Autodesk Inventor part; units mm, degrees
(part 3 of 3)
  line L456 (12.9282, 16.8333) -> (13.3502, 16.5006)
  line L457 (13.3502, 16.5006) -> (13.3076, 16.2984)
  line L458 (13.3076, 16.2984) -> (13.2446, 16.0331)
  line L459 (13.2446, 16.0331) -> (13.1744, 15.773)
  line L460 (13.1744, 15.773) -> (13.0968, 15.5182)
  line L461 (13.0968, 15.5182) -> (13.0115, 15.2694)
  line L462 (13.0115, 15.2694) -> (12.9181, 15.0268)
  line L463 (12.9181, 15.0268) -> (12.8161, 14.7913)
  line L464 (12.8161, 14.7913) -> (12.7045, 14.5637)
  line L465 (12.7045, 14.5637) -> (12.6447, 14.4533)
  line L466 (12.6447, 14.4533) -> (12.5818, 14.3456)
  line L467 (12.5818, 14.3456) -> (12.5153, 14.241)
  line L468 (12.5153, 14.241) -> (12.4803, 14.1901)
  line L469 (12.4803, 14.1901) -> (12.4439, 14.1406)
  line L470 (12.4439, 14.1406) -> (12.6143, 13.9062)
  line L471 (12.6143, 13.9062) -> (12.8737, 13.6665)
  line L472 (12.8737, 13.6665) -> (13.1207, 13.515)
  line L473 (13.1207, 13.515) -> (13.1672, 13.5552)
  line L474 (13.1672, 13.5552) -> (13.2151, 13.594)
  line L475 (13.2151, 13.594) -> (13.3142, 13.6686)
  line L476 (13.3142, 13.6686) -> (13.4166, 13.7397)
  line L477 (13.4166, 13.7397) -> (13.522, 13.808)
  line L478 (13.522, 13.808) -> (13.7402, 13.9371)
  line L479 (13.7402, 13.9371) -> (13.967, 14.0573)
  line L480 (13.967, 14.0573) -> (14.2014, 14.1694)
  line L481 (14.2014, 14.1694) -> (14.4428, 14.274)
  line L482 (14.4428, 14.274) -> (14.6907, 14.3714)
  line L483 (14.6907, 14.3714) -> (14.9445, 14.4617)
  line L484 (14.9445, 14.4617) -> (15.2041, 14.5453)
  line L485 (15.2041, 14.5453) -> (15.4023, 14.6036)
  line L486 (15.4023, 14.6036) -> (15.7671, 14.209)
  line L487 (15.7671, 14.209) -> (15.6934, 14.016)
  line L488 (15.6934, 14.016) -> (15.5897, 13.7638)
  line L489 (15.5897, 13.7638) -> (15.4797, 13.5178)
  line L490 (15.4797, 13.5178) -> (15.3632, 13.2784)
  line L491 (15.3632, 13.2784) -> (15.24, 13.0459)
  line L492 (15.24, 13.0459) -> (15.1098, 12.821)
  line L493 (15.1098, 12.821) -> (14.9722, 12.6043)
  line L494 (14.9722, 12.6043) -> (14.8264, 12.397)
  line L495 (14.8264, 12.397) -> (14.75, 12.2973)
  line L496 (14.75, 12.2973) -> (14.671, 12.2007)
  line L497 (14.671, 12.2007) -> (14.589, 12.1078)
  line L498 (14.589, 12.1078) -> (14.5465, 12.0631)
  line L499 (14.5465, 12.0631) -> (14.5028, 12.0199)
  line L500 (14.5028, 12.0199) -> (14.6344, 11.7617)
  line L501 (14.6344, 11.7617) -> (14.8531, 11.4843)
  line L502 (14.8531, 11.4843) -> (15.0734, 11.2961)
  line L503 (15.0734, 11.2961) -> (15.1256, 11.3285)
  line L504 (15.1256, 11.3285) -> (15.179, 11.3594)
  line L505 (15.179, 11.3594) -> (15.2885, 11.4175)
  line L506 (15.2885, 11.4175) -> (15.4008, 11.4717)
  line L507 (15.4008, 11.4717) -> (15.5156, 11.5227)
  line L508 (15.5156, 11.5227) -> (15.7512, 11.6161)
  line L509 (15.7512, 11.6161) -> (15.9941, 11.6993)
  line L510 (15.9941, 11.6993) -> (16.2432, 11.7734)
  line L511 (16.2432, 11.7734) -> (16.498, 11.8389)
  line L512 (16.498, 11.8389) -> (16.758, 11.8963)
  line L513 (16.758, 11.8963) -> (17.0229, 11.9459)
  line L514 (17.0229, 11.9459) -> (17.2923, 11.9878)
  line L515 (17.2923, 11.9878) -> (17.4972, 12.0144)
  line L516 (17.4972, 12.0144) -> (17.7957, 11.5676)
  line L517 (17.7957, 11.5676) -> (17.6928, 11.3885)
  line L518 (17.6928, 11.3885) -> (17.5509, 11.1556)
  line L519 (17.5509, 11.1556) -> (17.4037, 10.9299)
  line L520 (17.4037, 10.9299) -> (17.2512, 10.7116)
  line L521 (17.2512, 10.7116) -> (17.0932, 10.5012)
  line L522 (17.0932, 10.5012) -> (16.9294, 10.2995)
  line L523 (16.9294, 10.2995) -> (16.7596, 10.107)
  line L524 (16.7596, 10.107) -> (16.5831, 9.925)
  line L525 (16.5831, 9.925) -> (16.4921, 9.8385)
  line L526 (16.4921, 9.8385) -> (16.399, 9.7554)
  line L527 (16.399, 9.7554) -> (16.3034, 9.6765)
  line L528 (16.3034, 9.6765) -> (16.2545, 9.639)
  line L529 (16.2545, 9.639) -> (16.2045, 9.6031)
  line L530 (16.2045, 9.6031) -> (16.2942, 9.3276)
  line L531 (16.2942, 9.3276) -> (16.4668, 9.0194)
  line L532 (16.4668, 9.0194) -> (16.6549, 8.799)
  line L533 (16.6549, 8.799) -> (16.7115, 8.8229)
  line L534 (16.7115, 8.8229) -> (16.7691, 8.845)
  line L535 (16.7691, 8.845) -> (16.8863, 8.8853)
  line L536 (16.8863, 8.8853) -> (17.0058, 8.9213)
  line L537 (17.0058, 8.9213) -> (17.1271, 8.9537)
  line L538 (17.1271, 8.9537) -> (17.3745, 9.009)
  line L539 (17.3745, 9.009) -> (17.6273, 9.0533)
  line L540 (17.6273, 9.0533) -> (17.885, 9.0875)
  line L541 (17.885, 9.0875) -> (18.1469, 9.1123)
  line L542 (18.1469, 9.1123) -> (18.4127, 9.1283)
  line L543 (18.4127, 9.1283) -> (18.682, 9.1358)
  line L544 (18.682, 9.1358) -> (18.9547, 9.1351)
  line L545 (18.9547, 9.1351) -> (19.1612, 9.1293)
  line L546 (19.1612, 9.1293) -> (19.3862, 8.6413)
  line L547 (19.3862, 8.6413) -> (19.2565, 8.4805)
  line L548 (19.2565, 8.4805) -> (19.0799, 8.2727)
  line L549 (19.0799, 8.2727) -> (18.8993, 8.0727)
  line L550 (18.8993, 8.0727) -> (18.7145, 7.881)
  line L551 (18.7145, 7.881) -> (18.5255, 7.698)
  line L552 (18.5255, 7.698) -> (18.3322, 7.5243)
  line L553 (18.3322, 7.5243) -> (18.1343, 7.3608)
  line L554 (18.1343, 7.3608) -> (17.9316, 7.2086)
  line L555 (17.9316, 7.2086) -> (17.8282, 7.1374)
  line L556 (17.8282, 7.1374) -> (17.7232, 7.07)
  line L557 (17.7232, 7.07) -> (17.6165, 7.007)
  line L558 (17.6165, 7.007) -> (17.5622, 6.9776)
  line L559 (17.5622, 6.9776) -> (17.5073, 6.95)
  line L560 (17.5073, 6.95) -> (17.5527, 6.6638)
  line L561 (17.5527, 6.6638) -> (17.675, 6.3324)
  line L562 (17.675, 6.3324) -> (17.8263, 6.0853)
  line L563 (17.8263, 6.0853) -> (17.886, 6.1)
  line L564 (17.886, 6.1) -> (17.9463, 6.1128)
  line L565 (17.9463, 6.1128) -> (18.0684, 6.1343)
  line L566 (18.0684, 6.1343) -> (18.192, 6.1512)
  line L567 (18.192, 6.1512) -> (18.3169, 6.1642)
  line L568 (18.3169, 6.1642) -> (18.5699, 6.1802)
  line L569 (18.5699, 6.1802) -> (18.8265, 6.1843)
  line L570 (18.8265, 6.1843) -> (19.0863, 6.1778)
  line L571 (19.0863, 6.1778) -> (19.3489, 6.1613)
  line L572 (19.3489, 6.1613) -> (19.614, 6.1355)
  line L573 (19.614, 6.1355) -> (19.8812, 6.1008)
  line L574 (19.8812, 6.1008) -> (20.1504, 6.0575)
  line L575 (20.1504, 6.0575) -> (20.3535, 6.0194)
  line L576 (20.3535, 6.0194) -> (20.4993, 5.5022)
  line L577 (20.4993, 5.5022) -> (20.346, 5.3637)
  line L578 (20.346, 5.3637) -> (20.1392, 5.1861)
  line L579 (20.1392, 5.1861) -> (19.9295, 5.0169)
  line L580 (19.9295, 5.0169) -> (19.717, 4.8564)
  line L581 (19.717, 4.8564) -> (19.5017, 4.7052)
  line L582 (19.5017, 4.7052) -> (19.2836, 4.5639)
  line L583 (19.2836, 4.5639) -> (19.0626, 4.4333)
  line L584 (19.0626, 4.4333) -> (18.8385, 4.3147)
  line L585 (18.8385, 4.3147) -> (18.7252, 4.2606)
  line L586 (18.7252, 4.2606) -> (18.611, 4.2104)
  line L587 (18.611, 4.2104) -> (18.4957, 4.1649)
  line L588 (18.4957, 4.1649) -> (18.4376, 4.1443)
  line L589 (18.4376, 4.1443) -> (18.379, 4.1257)
  line L590 (18.379, 4.1257) -> (18.3791, 3.8359)
  line L591 (18.3791, 3.8359) -> (18.448, 3.4895)
  line L592 (18.448, 3.4895) -> (18.5588, 3.2217)
  line L593 (18.5588, 3.2217) -> (18.62, 3.2269)
  line L594 (18.62, 3.2269) -> (18.6816, 3.2301)
  line L595 (18.6816, 3.2301) -> (18.8056, 3.2322)
  line L596 (18.8056, 3.2322) -> (18.9303, 3.2296)
  line L597 (18.9303, 3.2296) -> (19.0557, 3.2229)
  line L598 (19.0557, 3.2229) -> (19.3081, 3.1991)
  line L599 (19.3081, 3.1991) -> (19.5622, 3.163)
  line L600 (19.5622, 3.163) -> (19.8178, 3.1159)
  line L601 (19.8178, 3.1159) -> (20.0745, 3.0586)
  line L602 (20.0745, 3.0586) -> (20.3323, 2.9917)
  line L603 (20.3323, 2.9917) -> (20.5908, 2.9156)
  line L604 (20.5908, 2.9156) -> (20.8499, 2.8307)
  line L605 (20.8499, 2.8307) -> (21.0445, 2.7613)
  line L606 (21.0445, 2.7613) -> (21.1077, 2.2277)
  line L607 (21.1077, 2.2277) -> (20.9346, 2.1148)
  line L608 (20.9346, 2.1148) -> (20.7025, 1.9718)
  line L609 (20.7025, 1.9718) -> (20.4689, 1.8374)
  line L610 (20.4689, 1.8374) -> (20.2339, 1.7122)
  line L611 (20.2339, 1.7122) -> (19.9976, 1.5965)
  line L612 (19.9976, 1.5965) -> (19.7601, 1.4911)
  line L613 (19.7601, 1.4911) -> (19.5214, 1.3967)
  line L614 (19.5214, 1.3967) -> (19.2815, 1.3146)
  line L615 (19.2815, 1.3146) -> (19.1612, 1.2789)
  line L616 (19.1612, 1.2789) -> (19.0405, 1.2472)
  line L617 (19.0405, 1.2472) -> (18.9195, 1.2203)
  line L618 (18.9195, 1.2203) -> (18.8589, 1.209)
  line L619 (18.8589, 1.209) -> (18.7981, 1.1998)
  line L620 (18.7981, 1.1998) -> (18.7529, 0.9135)
  line L621 (18.7529, 0.9135) -> (18.7667, 0.5606)
  line L622 (18.7667, 0.5606) -> (18.8343, 0.2788)
  line L623 (18.8343, 0.2788) -> (18.8956, 0.2744)
  line L624 (18.8956, 0.2744) -> (18.9569, 0.2679)
  line L625 (18.9569, 0.2679) -> (19.0797, 0.2506)
  line L626 (19.0797, 0.2506) -> (19.2024, 0.2285)
  line L627 (19.2024, 0.2285) -> (19.3252, 0.2022)
  line L628 (19.3252, 0.2022) -> (19.5708, 0.1393)
  line L629 (19.5708, 0.1393) -> (19.8162, 0.0639)
  line L630 (19.8162, 0.0639) -> (20.0612, -0.0226)
  line L631 (20.0612, -0.0226) -> (20.3059, -0.1194)
  line L632 (20.3059, -0.1194) -> (20.55, -0.2258)
  line L633 (20.55, -0.2258) -> (20.7934, -0.3414)
  line L634 (20.7934, -0.3414) -> (21.036, -0.4658)
  line L635 (21.036, -0.4658) -> (21.2174, -0.5647)
  line L636 (21.2174, -0.5647) -> (21.1963, -1.1017)
  line L637 (21.1963, -1.1017) -> (21.0077, -1.1861)
  line L638 (21.0077, -1.1861) -> (20.7561, -1.2911)
  line L639 (20.7561, -1.2911) -> (20.5043, -1.3872)
  line L640 (20.5043, -1.3872) -> (20.2526, -1.4742)
  line L641 (20.2526, -1.4742) -> (20.0012, -1.5514)
  line L642 (20.0012, -1.5514) -> (19.7501, -1.6184)
  line L643 (19.7501, -1.6184) -> (19.4995, -1.6743)
  line L644 (19.4995, -1.6743) -> (19.2498, -1.7179)
  line L645 (19.2498, -1.7179) -> (19.1253, -1.7343)
  line L646 (19.1253, -1.7343) -> (19.0012, -1.7468)
  line L647 (19.0012, -1.7468) -> (18.8775, -1.7544)
  line L648 (18.8775, -1.7544) -> (18.8158, -1.756)
  line L649 (18.8158, -1.756) -> (18.7543, -1.7557)
  line L650 (18.7543, -1.7557) -> (18.6649, -2.0313)
  line L651 (18.6649, -2.0313) -> (18.6234, -2.3821)
  line L652 (18.6234, -2.3821) -> (18.646, -2.6709)
  line L653 (18.646, -2.6709) -> (18.7059, -2.6849)
  line L654 (18.7059, -2.6849) -> (18.7655, -2.7009)
  line L655 (18.7655, -2.7009) -> (18.884, -2.7372)
  line L656 (18.884, -2.7372) -> (19.0018, -2.7783)
  line L657 (19.0018, -2.7783) -> (19.119, -2.8234)
  line L658 (19.119, -2.8234) -> (19.3516, -2.924)
  line L659 (19.3516, -2.924) -> (19.5822, -3.0368)
  line L660 (19.5822, -3.0368) -> (19.8107, -3.1606)
  line L661 (19.8107, -3.1606) -> (20.0372, -3.2944)
  line L662 (20.0372, -3.2944) -> (20.2616, -3.4377)
  line L663 (20.2616, -3.4377) -> (20.484, -3.59)
  line L664 (20.484, -3.59) -> (20.7042, -3.7508)
  line L665 (20.7042, -3.7508) -> (20.8678, -3.8769)
  line L666 (20.8678, -3.8769) -> (20.763, -4.404)
  line L667 (20.763, -4.404) -> (20.5635, -4.4578)
  line L668 (20.5635, -4.4578) -> (20.2986, -4.5222)
  line L669 (20.2986, -4.5222) -> (20.0349, -4.5777)
  line L670 (20.0349, -4.5777) -> (19.7727, -4.6242)
  line L671 (19.7727, -4.6242) -> (19.5122, -4.6612)
  line L672 (19.5122, -4.6612) -> (19.2537, -4.6881)
  line L673 (19.2537, -4.6881) -> (18.9975, -4.7041)
  line L674 (18.9975, -4.7041) -> (18.7441, -4.708)
  line L675 (18.7441, -4.708) -> (18.6186, -4.7049)
  line L676 (18.6186, -4.7049) -> (18.494, -4.6977)
  line L677 (18.494, -4.6977) -> (18.3706, -4.6859)
  line L678 (18.3706, -4.6859) -> (18.3095, -4.6779)
  line L679 (18.3095, -4.6779) -> (18.2488, -4.6679)
  line L680 (18.2488, -4.6679) -> (18.1173, -4.9261)
  line L681 (18.1173, -4.9261) -> (18.0215, -5.2661)
  line L682 (18.0215, -5.2661) -> (17.9986, -5.5549)
  line L683 (17.9986, -5.5549) -> (18.0556, -5.5781)
  line L684 (18.0556, -5.5781) -> (18.1119, -5.6032)
  line L685 (18.1119, -5.6032) -> (18.2233, -5.6576)
  line L686 (18.2233, -5.6576) -> (18.3332, -5.7166)
  line L687 (18.3332, -5.7166) -> (18.4419, -5.7795)
  line L688 (18.4419, -5.7795) -> (18.656, -5.9153)
  line L689 (18.656, -5.9153) -> (18.866, -6.0628)
  line L690 (18.866, -6.0628) -> (19.0724, -6.2208)
  line L691 (19.0724, -6.2208) -> (19.2751, -6.3884)
  line L692 (19.2751, -6.3884) -> (19.4744, -6.565)
  line L693 (19.4744, -6.565) -> (19.6702, -6.7502)
  line L694 (19.6702, -6.7502) -> (19.8625, -6.9435)
  line L695 (19.8625, -6.9435) -> (20.0044, -7.0936)
  line L696 (20.0044, -7.0936) -> (19.8184, -7.5978)
  line L697 (19.8184, -7.5978) -> (19.613, -7.6198)
  line L698 (19.613, -7.6198) -> (19.3412, -7.6419)
  line L699 (19.3412, -7.6419) -> (19.0721, -7.6555)
  line L700 (19.0721, -7.6555) -> (18.8059, -7.6604)
  line L701 (18.8059, -7.6604) -> (18.5428, -7.6562)
  line L702 (18.5428, -7.6562) -> (18.2833, -7.6423)
  line L703 (18.2833, -7.6423) -> (18.0278, -7.6181)
  line L704 (18.0278, -7.6181) -> (17.7768, -7.5823)
  line L705 (17.7768, -7.5823) -> (17.6533, -7.5595)
  line L706 (17.6533, -7.5595) -> (17.5314, -7.533)
  line L707 (17.5314, -7.533) -> (17.4114, -7.502)
  line L708 (17.4114, -7.502) -> (17.3523, -7.4845)
  line L709 (17.3523, -7.4845) -> (17.2939, -7.4652)
  line L710 (17.2939, -7.4652) -> (17.1237, -7.6996)
  line L711 (17.1237, -7.6996) -> (16.9758, -8.0204)
  line L712 (16.9758, -8.0204) -> (16.908, -8.3021)
  line L713 (16.908, -8.3021) -> (16.9606, -8.334)
  line L714 (16.9606, -8.334) -> (17.0124, -8.3676)
  line L715 (17.0124, -8.3676) -> (17.1139, -8.4387)
  line L716 (17.1139, -8.4387) -> (17.2132, -8.5142)
  line L717 (17.2132, -8.5142) -> (17.3107, -8.5933)
  line L718 (17.3107, -8.5933) -> (17.5009, -8.7609)
  line L719 (17.5009, -8.7609) -> (17.6853, -8.9394)
  line L720 (17.6853, -8.9394) -> (17.8644, -9.1278)
  line L721 (17.8644, -9.1278) -> (18.0385, -9.325)
  line L722 (18.0385, -9.325) -> (18.2076, -9.5307)
  line L723 (18.2076, -9.5307) -> (18.3721, -9.7442)
  line L724 (18.3721, -9.7442) -> (18.5318, -9.9652)
  line L725 (18.5318, -9.9652) -> (18.6484, -10.1357)
  line L726 (18.6484, -10.1357) -> (18.3859, -10.6045)
  line L727 (18.3859, -10.6045) -> (18.1795, -10.5941)
  line L728 (18.1795, -10.5941) -> (17.9077, -10.5734)
  line L729 (17.9077, -10.5734) -> (17.6397, -10.5448)
  line L730 (17.6397, -10.5448) -> (17.376, -10.508)
  line L731 (17.376, -10.508) -> (17.1168, -10.4627)
  line L732 (17.1168, -10.4627) -> (16.8627, -10.4084)
  line L733 (16.8627, -10.4084) -> (16.6141, -10.3444)
  line L734 (16.6141, -10.3444) -> (16.3718, -10.2698)
  line L735 (16.3718, -10.2698) -> (16.2534, -10.228)
  line L736 (16.2534, -10.228) -> (16.1372, -10.1828)
  line L737 (16.1372, -10.1828) -> (16.0235, -10.1334)
  line L738 (16.0235, -10.1334) -> (15.9678, -10.1068)
  line L739 (15.9678, -10.1068) -> (15.9132, -10.0786)
  line L740 (15.9132, -10.0786) -> (15.7083, -10.2836)
  line L741 (15.7083, -10.2836) -> (15.5121, -10.5773)
  line L742 (15.5121, -10.5773) -> (15.4011, -10.8449)
  line L743 (15.4011, -10.8449) -> (15.4481, -10.8846)
  line L744 (15.4481, -10.8846) -> (15.494, -10.9259)
  line L745 (15.494, -10.9259) -> (15.5831, -11.012)
  line L746 (15.5831, -11.012) -> (15.6694, -11.1021)
  line L747 (15.6694, -11.1021) -> (15.7533, -11.1955)
  line L748 (15.7533, -11.1955) -> (15.915, -11.3907)
  line L749 (15.915, -11.3907) -> (16.0692, -11.596)
  line L750 (16.0692, -11.596) -> (16.2166, -11.81)
  line L751 (16.2166, -11.81) -> (16.3576, -12.0321)
  line L752 (16.3576, -12.0321) -> (16.4926, -12.2616)
  line L753 (16.4926, -12.2616) -> (16.6215, -12.4982)
  line L754 (16.6215, -12.4982) -> (16.7447, -12.7415)
  line L755 (16.7447, -12.7415) -> (16.8333, -12.9281)
  line L756 (16.8333, -12.9281) -> (16.5006, -13.3502)
  line L757 (16.5006, -13.3502) -> (16.2984, -13.3076)
  line L758 (16.2984, -13.3076) -> (16.0331, -13.2446)
  line L759 (16.0331, -13.2446) -> (15.773, -13.1744)
  line L760 (15.773, -13.1744) -> (15.5182, -13.0968)
  line L761 (15.5182, -13.0968) -> (15.2694, -13.0115)
  line L762 (15.2694, -13.0115) -> (15.0268, -12.9181)
  line L763 (15.0268, -12.9181) -> (14.7913, -12.8161)
  line L764 (14.7913, -12.8161) -> (14.5637, -12.7045)
  line L765 (14.5637, -12.7045) -> (14.4533, -12.6447)
  line L766 (14.4533, -12.6447) -> (14.3456, -12.5818)
  line L767 (14.3456, -12.5818) -> (14.241, -12.5153)
  line L768 (14.241, -12.5153) -> (14.1901, -12.4803)
  line L769 (14.1901, -12.4803) -> (14.1406, -12.4439)
  line L770 (14.1406, -12.4439) -> (13.9062, -12.6143)
  line L771 (13.9062, -12.6143) -> (13.6665, -12.8737)
  line L772 (13.6665, -12.8737) -> (13.515, -13.1207)
  line L773 (13.515, -13.1207) -> (13.5552, -13.1672)
  line L774 (13.5552, -13.1672) -> (13.594, -13.2151)
  line L775 (13.594, -13.2151) -> (13.6686, -13.3142)
  line L776 (13.6686, -13.3142) -> (13.7397, -13.4166)
  line L777 (13.7397, -13.4166) -> (13.808, -13.522)
  line L778 (13.808, -13.522) -> (13.9371, -13.7402)
  line L779 (13.9371, -13.7402) -> (14.0573, -13.967)
  line L780 (14.0573, -13.967) -> (14.1694, -14.2014)
  line L781 (14.1694, -14.2014) -> (14.274, -14.4428)
  line L782 (14.274, -14.4428) -> (14.3714, -14.6907)
  line L783 (14.3714, -14.6907) -> (14.4617, -14.9445)
  line L784 (14.4617, -14.9445) -> (14.5453, -15.2041)
  line L785 (14.5453, -15.2041) -> (14.6036, -15.4023)
  line L786 (14.6036, -15.4023) -> (14.209, -15.7671)
  line L787 (14.209, -15.7671) -> (14.016, -15.6934)
  line L788 (14.016, -15.6934) -> (13.7638, -15.5897)
  line L789 (13.7638, -15.5897) -> (13.5178, -15.4797)
  line L790 (13.5178, -15.4797) -> (13.2784, -15.3632)
  line L791 (13.2784, -15.3632) -> (13.0459, -15.24)
  line L792 (13.0459, -15.24) -> (12.821, -15.1098)
  line L793 (12.821, -15.1098) -> (12.6043, -14.9722)
  line L794 (12.6043, -14.9722) -> (12.397, -14.8264)
  line L795 (12.397, -14.8264) -> (12.2973, -14.75)
  line L796 (12.2973, -14.75) -> (12.2007, -14.671)
  line L797 (12.2007, -14.671) -> (12.1078, -14.589)
  line L798 (12.1078, -14.589) -> (12.0631, -14.5465)
  line L799 (12.0631, -14.5465) -> (12.0199, -14.5028)
  line L800 (12.0199, -14.5028) -> (11.7617, -14.6344)
  line L801 (11.7617, -14.6344) -> (11.4843, -14.8531)
  line L802 (11.4843, -14.8531) -> (11.2961, -15.0734)
  line L803 (11.2961, -15.0734) -> (11.3285, -15.1256)
  line L804 (11.3285, -15.1256) -> (11.3594, -15.179)
  line L805 (11.3594, -15.179) -> (11.4175, -15.2885)
  line L806 (11.4175, -15.2885) -> (11.4717, -15.4008)
  line L807 (11.4717, -15.4008) -> (11.5227, -15.5156)
  line L808 (11.5227, -15.5156) -> (11.6161, -15.7512)
  line L809 (11.6161, -15.7512) -> (11.6993, -15.9941)
  line L810 (11.6993, -15.9941) -> (11.7734, -16.2432)
  line L811 (11.7734, -16.2432) -> (11.8389, -16.498)
  line L812 (11.8389, -16.498) -> (11.8963, -16.758)
  line L813 (11.8963, -16.758) -> (11.9458, -17.0229)
  line L814 (11.9458, -17.0229) -> (11.9878, -17.2923)
  line L815 (11.9878, -17.2923) -> (12.0144, -17.4972)
  line L816 (12.0144, -17.4972) -> (11.5676, -17.7957)
  line L817 (11.5676, -17.7957) -> (11.3885, -17.6928)
  line L818 (11.3885, -17.6928) -> (11.1556, -17.5509)
  line L819 (11.1556, -17.5509) -> (10.9298, -17.4037)
  line L820 (10.9298, -17.4037) -> (10.7116, -17.2512)
  line L821 (10.7116, -17.2512) -> (10.5012, -17.0932)
  line L822 (10.5012, -17.0932) -> (10.2995, -16.9294)
  line L823 (10.2995, -16.9294) -> (10.107, -16.7596)
  line L824 (10.107, -16.7596) -> (9.925, -16.5831)
  line L825 (9.925, -16.5831) -> (9.8385, -16.4921)
  line L826 (9.8385, -16.4921) -> (9.7554, -16.399)
  line L827 (9.7554, -16.399) -> (9.6765, -16.3034)
  line L828 (9.6765, -16.3034) -> (9.639, -16.2545)
  line L829 (9.639, -16.2545) -> (9.6031, -16.2045)
  line L830 (9.6031, -16.2045) -> (9.3276, -16.2942)
  line L831 (9.3276, -16.2942) -> (9.0194, -16.4668)
  line L832 (9.0194, -16.4668) -> (8.799, -16.6549)
  line L833 (8.799, -16.6549) -> (8.8229, -16.7115)
  line L834 (8.8229, -16.7115) -> (8.845, -16.7691)
  line L835 (8.845, -16.7691) -> (8.8853, -16.8863)
  line L836 (8.8853, -16.8863) -> (8.9213, -17.0058)
  line L837 (8.9213, -17.0058) -> (8.9537, -17.1271)
  line L838 (8.9537, -17.1271) -> (9.009, -17.3745)
  line L839 (9.009, -17.3745) -> (9.0533, -17.6273)
  line L840 (9.0533, -17.6273) -> (9.0875, -17.885)
  line L841 (9.0875, -17.885) -> (9.1123, -18.1469)
  line L842 (9.1123, -18.1469) -> (9.1283, -18.4127)
  line L843 (9.1283, -18.4127) -> (9.1358, -18.682)
  line L844 (9.1358, -18.682) -> (9.1351, -18.9547)
  line L845 (9.1351, -18.9547) -> (9.1293, -19.1612)
  line L846 (9.1293, -19.1612) -> (8.6413, -19.3862)
  line L847 (8.6413, -19.3862) -> (8.4805, -19.2565)
  line L848 (8.4805, -19.2565) -> (8.2727, -19.0799)
  line L849 (8.2727, -19.0799) -> (8.0727, -18.8993)
  line L850 (8.0727, -18.8993) -> (7.881, -18.7145)
  line L851 (7.881, -18.7145) -> (7.698, -18.5255)
  line L852 (7.698, -18.5255) -> (7.5243, -18.3322)
  line L853 (7.5243, -18.3322) -> (7.3607, -18.1343)
  line L854 (7.3607, -18.1343) -> (7.2086, -17.9316)
  line L855 (7.2086, -17.9316) -> (7.1374, -17.8282)
  line L856 (7.1374, -17.8282) -> (7.07, -17.7232)
  line L857 (7.07, -17.7232) -> (7.007, -17.6165)
  line L858 (7.007, -17.6165) -> (6.9776, -17.5622)
  line L859 (6.9776, -17.5622) -> (6.95, -17.5073)
  line L860 (6.95, -17.5073) -> (6.6638, -17.5527)
  line L861 (6.6638, -17.5527) -> (6.3324, -17.675)
  line L862 (6.3324, -17.675) -> (6.0853, -17.8263)
  line L863 (6.0853, -17.8263) -> (6.1, -17.886)
  line L864 (6.1, -17.886) -> (6.1128, -17.9463)
  line L865 (6.1128, -17.9463) -> (6.1343, -18.0684)
  line L866 (6.1343, -18.0684) -> (6.1512, -18.192)
  line L867 (6.1512, -18.192) -> (6.1642, -18.3169)
  line L868 (6.1642, -18.3169) -> (6.1802, -18.5699)
  line L869 (6.1802, -18.5699) -> (6.1843, -18.8265)
  line L870 (6.1843, -18.8265) -> (6.1778, -19.0864)
  line L871 (6.1778, -19.0864) -> (6.1613, -19.3489)
  line L872 (6.1613, -19.3489) -> (6.1355, -19.614)
  line L873 (6.1355, -19.614) -> (6.1008, -19.8812)
  line L874 (6.1008, -19.8812) -> (6.0575, -20.1504)
  line L875 (6.0575, -20.1504) -> (6.0194, -20.3535)
  line L876 (6.0194, -20.3535) -> (5.5022, -20.4993)
  line L877 (5.5022, -20.4993) -> (5.3637, -20.346)
  line L878 (5.3637, -20.346) -> (5.1861, -20.1392)
  line L879 (5.1861, -20.1392) -> (5.0168, -19.9295)
  line L880 (5.0168, -19.9295) -> (4.8564, -19.717)
  line L881 (4.8564, -19.717) -> (4.7052, -19.5017)
  line L882 (4.7052, -19.5017) -> (4.5639, -19.2836)
  line L883 (4.5639, -19.2836) -> (4.4333, -19.0626)
  line L884 (4.4333, -19.0626) -> (4.3147, -18.8385)
  line L885 (4.3147, -18.8385) -> (4.2606, -18.7252)
  line L886 (4.2606, -18.7252) -> (4.2104, -18.611)
  line L887 (4.2104, -18.611) -> (4.1649, -18.4957)
  line L888 (4.1649, -18.4957) -> (4.1443, -18.4376)
  line L889 (4.1443, -18.4376) -> (4.1256, -18.379)
  line L890 (4.1256, -18.379) -> (3.8359, -18.3791)
  line L891 (3.8359, -18.3791) -> (3.4895, -18.448)
  line L892 (3.4895, -18.448) -> (3.2217, -18.5588)
  line L893 (3.2217, -18.5588) -> (3.2269, -18.62)
  line L894 (3.2269, -18.62) -> (3.2301, -18.6816)
  line L895 (3.2301, -18.6816) -> (3.2322, -18.8056)
  line L896 (3.2322, -18.8056) -> (3.2296, -18.9303)
  line L897 (3.2296, -18.9303) -> (3.2229, -19.0557)
  line L898 (3.2229, -19.0557) -> (3.1991, -19.3081)
  line L899 (3.1991, -19.3081) -> (3.163, -19.5622)
  line L900 (3.163, -19.5622) -> (3.1159, -19.8178)
  line L901 (3.1159, -19.8178) -> (3.0586, -20.0746)
  line L902 (3.0586, -20.0746) -> (2.9917, -20.3323)
  line L903 (2.9917, -20.3323) -> (2.9156, -20.5908)
  line L904 (2.9156, -20.5908) -> (2.8307, -20.8499)
  line L905 (2.8307, -20.8499) -> (2.7613, -21.0445)
  line L906 (2.7613, -21.0445) -> (2.2277, -21.1077)
  line L907 (2.2277, -21.1077) -> (2.1148, -20.9346)
  line L908 (2.1148, -20.9346) -> (1.9718, -20.7025)
  line L909 (1.9718, -20.7025) -> (1.8374, -20.4689)
  line L910 (1.8374, -20.4689) -> (1.7122, -20.2339)
  line L911 (1.7122, -20.2339) -> (1.5965, -19.9976)
  line L912 (1.5965, -19.9976) -> (1.4911, -19.7601)
  line L913 (1.4911, -19.7601) -> (1.3967, -19.5214)
  line L914 (1.3967, -19.5214) -> (1.3146, -19.2815)
  line L915 (1.3146, -19.2815) -> (1.2789, -19.1612)
  line L916 (1.2789, -19.1612) -> (1.2472, -19.0405)
  line L917 (1.2472, -19.0405) -> (1.2203, -18.9195)
  line L918 (1.2203, -18.9195) -> (1.209, -18.8589)
  line L919 (1.209, -18.8589) -> (1.1998, -18.7981)
  line L920 (1.1998, -18.7981) -> (0.9135, -18.7529)
  line L921 (0.9135, -18.7529) -> (0.5606, -18.7667)
  line L922 (0.5606, -18.7667) -> (0.2788, -18.8343)
  line L923 (0.2788, -18.8343) -> (0.2744, -18.8956)
  line L924 (0.2744, -18.8956) -> (0.2679, -18.9569)
  line L925 (0.2679, -18.9569) -> (0.2506, -19.0797)
  line L926 (0.2506, -19.0797) -> (0.2285, -19.2025)
  line L927 (0.2285, -19.2025) -> (0.2022, -19.3252)
  line L928 (0.2022, -19.3252) -> (0.1393, -19.5708)
  line L929 (0.1393, -19.5708) -> (0.0639, -19.8162)
  line L930 (0.0639, -19.8162) -> (-0.0226, -20.0612)
  line L931 (-0.0226, -20.0612) -> (-0.1194, -20.3059)
  line L932 (-0.1194, -20.3059) -> (-0.2258, -20.55)
  line L933 (-0.2258, -20.55) -> (-0.3414, -20.7934)
  line L934 (-0.3414, -20.7934) -> (-0.4658, -21.036)
  line L935 (-0.4658, -21.036) -> (-0.5647, -21.2174)
  line L936 (-0.5647, -21.2174) -> (-1.1017, -21.1963)
  line L937 (-1.1017, -21.1963) -> (-1.1861, -21.0077)
  line L938 (-1.1861, -21.0077) -> (-1.2911, -20.7561)
  line L939 (-1.2911, -20.7561) -> (-1.3872, -20.5043)
  line L940 (-1.3872, -20.5043) -> (-1.4742, -20.2526)
  line L941 (-1.4742, -20.2526) -> (-1.5514, -20.0012)
  line L942 (-1.5514, -20.0012) -> (-1.6184, -19.7501)
  line L943 (-1.6184, -19.7501) -> (-1.6743, -19.4995)
  line L944 (-1.6743, -19.4995) -> (-1.7179, -19.2498)
  line L945 (-1.7179, -19.2498) -> (-1.7343, -19.1253)
  line L946 (-1.7343, -19.1253) -> (-1.7468, -19.0012)
  line L947 (-1.7468, -19.0012) -> (-1.7544, -18.8775)
  line L948 (-1.7544, -18.8775) -> (-1.756, -18.8158)
  line L949 (-1.756, -18.8158) -> (-1.7557, -18.7543)
  line L950 (-1.7557, -18.7543) -> (-2.0313, -18.6649)
  line L951 (-2.0313, -18.6649) -> (-2.3821, -18.6234)
  line L952 (-2.3821, -18.6234) -> (-2.6709, -18.646)
  line L953 (-2.6709, -18.646) -> (-2.6849, -18.7059)
  line L954 (-2.6849, -18.7059) -> (-2.7009, -18.7654)
  line L955 (-2.7009, -18.7654) -> (-2.7372, -18.884)
  line L956 (-2.7372, -18.884) -> (-2.7783, -19.0018)
  line L957 (-2.7783, -19.0018) -> (-2.8234, -19.119)
  line L958 (-2.8234, -19.119) -> (-2.924, -19.3516)
  line L959 (-2.924, -19.3516) -> (-3.0368, -19.5822)
  line L960 (-3.0368, -19.5822) -> (-3.1606, -19.8107)
  line L961 (-3.1606, -19.8107) -> (-3.2944, -20.0372)
  line L962 (-3.2944, -20.0372) -> (-3.4377, -20.2616)
  line L963 (-3.4377, -20.2616) -> (-3.59, -20.484)
  line L964 (-3.59, -20.484) -> (-3.7508, -20.7042)
  line L965 (-3.7508, -20.7042) -> (-3.8769, -20.8678)
  line L966 (-3.8769, -20.8678) -> (-4.404, -20.763)
  line L967 (-4.404, -20.763) -> (-4.4578, -20.5635)
  line L968 (-4.4578, -20.5635) -> (-4.5222, -20.2986)
  line L969 (-4.5222, -20.2986) -> (-4.5777, -20.0349)
  line L970 (-4.5777, -20.0349) -> (-4.6242, -19.7727)
  line L971 (-4.6242, -19.7727) -> (-4.6612, -19.5122)
  line L972 (-4.6612, -19.5122) -> (-4.6881, -19.2537)
  line L973 (-4.6881, -19.2537) -> (-4.7041, -18.9975)
  line L974 (-4.7041, -18.9975) -> (-4.708, -18.7441)
  line L975 (-4.708, -18.7441) -> (-4.7049, -18.6186)
  line L976 (-4.7049, -18.6186) -> (-4.6977, -18.494)
  line L977 (-4.6977, -18.494) -> (-4.6859, -18.3706)
  line L978 (-4.6859, -18.3706) -> (-4.6779, -18.3095)
  line L979 (-4.6779, -18.3095) -> (-4.6679, -18.2488)
  line L980 (-4.6679, -18.2488) -> (-4.9261, -18.1173)
  line L981 (-4.9261, -18.1173) -> (-5.2661, -18.0214)
  line L982 (-5.2661, -18.0214) -> (-5.5549, -17.9986)
  line L983 (-5.5549, -17.9986) -> (-5.5781, -18.0556)
  line L984 (-5.5781, -18.0556) -> (-5.6032, -18.1119)
  line L985 (-5.6032, -18.1119) -> (-5.6576, -18.2233)
  line L986 (-5.6576, -18.2233) -> (-5.7166, -18.3332)
  line L987 (-5.7166, -18.3332) -> (-5.7795, -18.4419)
  line L988 (-5.7795, -18.4419) -> (-5.9153, -18.656)
  line L989 (-5.9153, -18.656) -> (-6.0628, -18.866)
  line L990 (-6.0628, -18.866) -> (-6.2208, -19.0724)
  line L991 (-6.2208, -19.0724) -> (-6.3884, -19.2751)
  line L992 (-6.3884, -19.2751) -> (-6.565, -19.4744)
  line L993 (-6.565, -19.4744) -> (-6.7502, -19.6702)
  line L994 (-6.7502, -19.6702) -> (-6.9435, -19.8625)
  line L995 (-6.9435, -19.8625) -> (-7.0936, -20.0044)
  line L996 (-7.0936, -20.0044) -> (-7.5978, -19.8184)
  line L997 (-7.5978, -19.8184) -> (-7.6198, -19.613)
  line L998 (-7.6198, -19.613) -> (-7.6419, -19.3412)
  line L999 (-7.6419, -19.3412) -> (-7.6555, -19.0721)
  line L1000 (-7.6555, -19.0721) -> (-7.6604, -18.8059)
  line L1001 (-7.6604, -18.8059) -> (-7.6562, -18.5428)
  line L1002 (-7.6562, -18.5428) -> (-7.6423, -18.2833)
  line L1003 (-7.6423, -18.2833) -> (-7.6181, -18.0278)
  line L1004 (-7.6181, -18.0278) -> (-7.5823, -17.7768)
  line L1005 (-7.5823, -17.7768) -> (-7.5595, -17.6533)
  line L1006 (-7.5595, -17.6533) -> (-7.533, -17.5314)
  line L1007 (-7.533, -17.5314) -> (-7.502, -17.4114)
  line L1008 (-7.502, -17.4114) -> (-7.4845, -17.3523)
  line L1009 (-7.4845, -17.3523) -> (-7.4652, -17.2939)
  line L1010 (-7.4652, -17.2939) -> (-7.6996, -17.1237)
  line L1011 (-7.6996, -17.1237) -> (-8.0204, -16.9758)
  line L1012 (-8.0204, -16.9758) -> (-8.3021, -16.908)
  line L1013 (-8.3021, -16.908) -> (-8.334, -16.9607)
  line L1014 (-8.334, -16.9607) -> (-8.3676, -17.0124)
  line L1015 (-8.3676, -17.0124) -> (-8.4387, -17.1139)
  line L1016 (-8.4387, -17.1139) -> (-8.5142, -17.2132)
  line L1017 (-8.5142, -17.2132) -> (-8.5933, -17.3107)
  line L1018 (-8.5933, -17.3107) -> (-8.7609, -17.5009)
  line L1019 (-8.7609, -17.5009) -> (-8.9394, -17.6853)
  line L1020 (-8.9394, -17.6853) -> (-9.1278, -17.8644)
  line L1021 (-9.1278, -17.8644) -> (-9.325, -18.0385)
  line L1022 (-9.325, -18.0385) -> (-9.5307, -18.2076)
  line L1023 (-9.5307, -18.2076) -> (-9.7442, -18.3721)
  line L1024 (-9.7442, -18.3721) -> (-9.9652, -18.5317)
  line L1025 (-9.9652, -18.5317) -> (-10.1357, -18.6484)
  line L1026 (-10.1357, -18.6484) -> (-10.6045, -18.3859)
  line L1027 (-10.6045, -18.3859) -> (-10.5941, -18.1795)
  line L1028 (-10.5941, -18.1795) -> (-10.5734, -17.9077)
  line L1029 (-10.5734, -17.9077) -> (-10.5448, -17.6397)
  line L1030 (-10.5448, -17.6397) -> (-10.508, -17.376)
  line L1031 (-10.508, -17.376) -> (-10.4627, -17.1168)
  line L1032 (-10.4627, -17.1168) -> (-10.4084, -16.8627)
  line L1033 (-10.4084, -16.8627) -> (-10.3444, -16.6141)
  line L1034 (-10.3444, -16.6141) -> (-10.2698, -16.3718)
  line L1035 (-10.2698, -16.3718) -> (-10.228, -16.2534)
  line L1036 (-10.228, -16.2534) -> (-10.1828, -16.1372)
  line L1037 (-10.1828, -16.1372) -> (-10.1334, -16.0235)
  line L1038 (-10.1334, -16.0235) -> (-10.1068, -15.9678)
  line L1039 (-10.1068, -15.9678) -> (-10.0786, -15.9132)
  line L1040 (-10.0786, -15.9132) -> (-10.2836, -15.7083)
  line L1041 (-10.2836, -15.7083) -> (-10.5773, -15.5121)
  line L1042 (-10.5773, -15.5121) -> (-10.8449, -15.4011)
  line L1043 (-10.8449, -15.4011) -> (-10.8846, -15.4481)
  line L1044 (-10.8846, -15.4481) -> (-10.9259, -15.494)
  line L1045 (-10.9259, -15.494) -> (-11.012, -15.5831)
  line L1046 (-11.012, -15.5831) -> (-11.1021, -15.6694)
  line L1047 (-11.1021, -15.6694) -> (-11.1955, -15.7533)
  line L1048 (-11.1955, -15.7533) -> (-11.3908, -15.915)
  line L1049 (-11.3908, -15.915) -> (-11.596, -16.0692)
  line L1050 (-11.596, -16.0692) -> (-11.81, -16.2166)
  line L1051 (-11.81, -16.2166) -> (-12.0321, -16.3576)
  line L1052 (-12.0321, -16.3576) -> (-12.2616, -16.4926)
  line L1053 (-12.2616, -16.4926) -> (-12.4982, -16.6215)
  line L1054 (-12.4982, -16.6215) -> (-12.7415, -16.7447)
  line L1055 (-12.7415, -16.7447) -> (-12.9282, -16.8333)
  line L1056 (-12.9282, -16.8333) -> (-13.3502, -16.5006)
  line L1057 (-13.3502, -16.5006) -> (-13.3076, -16.2984)
  line L1058 (-13.3076, -16.2984) -> (-13.2446, -16.0331)
  line L1059 (-13.2446, -16.0331) -> (-13.1744, -15.773)
  line L1060 (-13.1744, -15.773) -> (-13.0968, -15.5182)
  line L1061 (-13.0968, -15.5182) -> (-13.0115, -15.2694)
  line L1062 (-13.0115, -15.2694) -> (-12.9181, -15.0268)
  line L1063 (-12.9181, -15.0268) -> (-12.8161, -14.7913)
  line L1064 (-12.8161, -14.7913) -> (-12.7045, -14.5637)
  line L1065 (-12.7045, -14.5637) -> (-12.6447, -14.4533)
  line L1066 (-12.6447, -14.4533) -> (-12.5818, -14.3456)
  line L1067 (-12.5818, -14.3456) -> (-12.5153, -14.241)
  line L1068 (-12.5153, -14.241) -> (-12.4803, -14.1901)
  line L1069 (-12.4803, -14.1901) -> (-12.4439, -14.1406)
  line L1070 (-12.4439, -14.1406) -> (-12.6143, -13.9062)
  line L1071 (-12.6143, -13.9062) -> (-12.8737, -13.6665)
  line L1072 (-12.8737, -13.6665) -> (-13.1207, -13.515)
  line L1073 (-13.1207, -13.515) -> (-13.1672, -13.5552)
  line L1074 (-13.1672, -13.5552) -> (-13.2151, -13.594)
  line L1075 (-13.2151, -13.594) -> (-13.3142, -13.6686)
  line L1076 (-13.3142, -13.6686) -> (-13.4166, -13.7397)
  line L1077 (-13.4166, -13.7397) -> (-13.522, -13.808)
  line L1078 (-13.522, -13.808) -> (-13.7402, -13.9371)
  line L1079 (-13.7402, -13.9371) -> (-13.967, -14.0573)
  line L1080 (-13.967, -14.0573) -> (-14.2014, -14.1694)
  line L1081 (-14.2014, -14.1694) -> (-14.4428, -14.274)
  line L1082 (-14.4428, -14.274) -> (-14.6907, -14.3714)
  line L1083 (-14.6907, -14.3714) -> (-14.9445, -14.4617)
  line L1084 (-14.9445, -14.4617) -> (-15.2041, -14.5453)
  line L1085 (-15.2041, -14.5453) -> (-15.4023, -14.6036)
  line L1086 (-15.4023, -14.6036) -> (-15.7671, -14.209)
  line L1087 (-15.7671, -14.209) -> (-15.6934, -14.016)
  line L1088 (-15.6934, -14.016) -> (-15.5897, -13.7638)
  line L1089 (-15.5897, -13.7638) -> (-15.4797, -13.5178)
  line L1090 (-15.4797, -13.5178) -> (-15.3632, -13.2784)
  line L1091 (-15.3632, -13.2784) -> (-15.24, -13.0459)
  line L1092 (-15.24, -13.0459) -> (-15.1098, -12.821)
  line L1093 (-15.1098, -12.821) -> (-14.9722, -12.6043)
  line L1094 (-14.9722, -12.6043) -> (-14.8264, -12.397)
  line L1095 (-14.8264, -12.397) -> (-14.75, -12.2973)
  line L1096 (-14.75, -12.2973) -> (-14.671, -12.2007)
  line L1097 (-14.671, -12.2007) -> (-14.589, -12.1078)
  line L1098 (-14.589, -12.1078) -> (-14.5465, -12.0631)
  line L1099 (-14.5465, -12.0631) -> (-14.5028, -12.0199)
  line L1100 (-14.5028, -12.0199) -> (-14.6344, -11.7617)
  line L1101 (-14.6344, -11.7617) -> (-14.8531, -11.4843)
  line L1102 (-14.8531, -11.4843) -> (-15.0734, -11.2961)
  line L1103 (-15.0734, -11.2961) -> (-15.1256, -11.3285)
  line L1104 (-15.1256, -11.3285) -> (-15.179, -11.3594)
  line L1105 (-15.179, -11.3594) -> (-15.2885, -11.4175)
  line L1106 (-15.2885, -11.4175) -> (-15.4008, -11.4717)
  line L1107 (-15.4008, -11.4717) -> (-15.5156, -11.5227)
  line L1108 (-15.5156, -11.5227) -> (-15.7512, -11.6161)
  line L1109 (-15.7512, -11.6161) -> (-15.9941, -11.6993)
  line L1110 (-15.9941, -11.6993) -> (-16.2432, -11.7734)
  line L1111 (-16.2432, -11.7734) -> (-16.498, -11.8389)
  line L1112 (-16.498, -11.8389) -> (-16.758, -11.8963)
  line L1113 (-16.758, -11.8963) -> (-17.0229, -11.9459)
  line L1114 (-17.0229, -11.9459) -> (-17.2923, -11.9878)
  line L1115 (-17.2923, -11.9878) -> (-17.4972, -12.0144)
  line L1116 (-17.4972, -12.0144) -> (-17.7957, -11.5676)
  line L1117 (-17.7957, -11.5676) -> (-17.6928, -11.3885)
  line L1118 (-17.6928, -11.3885) -> (-17.5509, -11.1556)
  line L1119 (-17.5509, -11.1556) -> (-17.4038, -10.9299)
  line L1120 (-17.4038, -10.9299) -> (-17.2512, -10.7116)
  line L1121 (-17.2512, -10.7116) -> (-17.0932, -10.5012)
  line L1122 (-17.0932, -10.5012) -> (-16.9294, -10.2994)
  line L1123 (-16.9294, -10.2994) -> (-16.7596, -10.107)
  line L1124 (-16.7596, -10.107) -> (-16.5831, -9.925)
  line L1125 (-16.5831, -9.925) -> (-16.4921, -9.8385)
  line L1126 (-16.4921, -9.8385) -> (-16.399, -9.7554)
  line L1127 (-16.399, -9.7554) -> (-16.3034, -9.6765)
  line L1128 (-16.3034, -9.6765) -> (-16.2545, -9.639)
  line L1129 (-16.2545, -9.639) -> (-16.2045, -9.6031)
  line L1130 (-16.2045, -9.6031) -> (-16.2942, -9.3276)
  line L1131 (-16.2942, -9.3276) -> (-16.4668, -9.0194)
  line L1132 (-16.4668, -9.0194) -> (-16.6549, -8.799)
  line L1133 (-16.6549, -8.799) -> (-16.7115, -8.8229)
  line L1134 (-16.7115, -8.8229) -> (-16.7691, -8.845)
  line L1135 (-16.7691, -8.845) -> (-16.8864, -8.8853)
  line L1136 (-16.8864, -8.8853) -> (-17.0058, -8.9213)
  line L1137 (-17.0058, -8.9213) -> (-17.1271, -8.9537)
  line L1138 (-17.1271, -8.9537) -> (-17.3745, -9.009)
  line L1139 (-17.3745, -9.009) -> (-17.6273, -9.0533)
  line L1140 (-17.6273, -9.0533) -> (-17.885, -9.0875)
  line L1141 (-17.885, -9.0875) -> (-18.1469, -9.1123)
  line L1142 (-18.1469, -9.1123) -> (-18.4127, -9.1283)
  line L1143 (-18.4127, -9.1283) -> (-18.682, -9.1358)
  line L1144 (-18.682, -9.1358) -> (-18.9547, -9.1351)
  line L1145 (-18.9547, -9.1351) -> (-19.1612, -9.1293)
  line L1146 (-19.1612, -9.1293) -> (-19.3862, -8.6413)
  line L1147 (-19.3862, -8.6413) -> (-19.2565, -8.4805)
  line L1148 (-19.2565, -8.4805) -> (-19.0799, -8.2727)
  line L1149 (-19.0799, -8.2727) -> (-18.8993, -8.0727)
  line L1150 (-18.8993, -8.0727) -> (-18.7145, -7.881)
  line L1151 (-18.7145, -7.881) -> (-18.5255, -7.698)
  line L1152 (-18.5255, -7.698) -> (-18.3322, -7.5243)
  line L1153 (-18.3322, -7.5243) -> (-18.1343, -7.3608)
  line L1154 (-18.1343, -7.3608) -> (-17.9316, -7.2086)
  line L1155 (-17.9316, -7.2086) -> (-17.8282, -7.1374)
  line L1156 (-17.8282, -7.1374) -> (-17.7232, -7.07)
  line L1157 (-17.7232, -7.07) -> (-17.6165, -7.007)
  line L1158 (-17.6165, -7.007) -> (-17.5622, -6.9776)
  line L1159 (-17.5622, -6.9776) -> (-17.5073, -6.95)
  line L1160 (-17.5073, -6.95) -> (-17.5527, -6.6638)
  line L1161 (-17.5527, -6.6638) -> (-17.675, -6.3324)
  line L1162 (-17.675, -6.3324) -> (-17.8263, -6.0853)
  line L1163 (-17.8263, -6.0853) -> (-17.886, -6.1)
  line L1164 (-17.886, -6.1) -> (-17.9463, -6.1128)
  line L1165 (-17.9463, -6.1128) -> (-18.0684, -6.1343)
  line L1166 (-18.0684, -6.1343) -> (-18.192, -6.1512)
  line L1167 (-18.192, -6.1512) -> (-18.3169, -6.1642)
  line L1168 (-18.3169, -6.1642) -> (-18.5699, -6.1802)
  line L1169 (-18.5699, -6.1802) -> (-18.8265, -6.1843)
  line L1170 (-18.8265, -6.1843) -> (-19.0864, -6.1778)
  line L1171 (-19.0864, -6.1778) -> (-19.3489, -6.1613)
  line L1172 (-19.3489, -6.1613) -> (-19.614, -6.1355)
  line L1173 (-19.614, -6.1355) -> (-19.8812, -6.1008)
  line L1174 (-19.8812, -6.1008) -> (-20.1504, -6.0575)
  line L1175 (-20.1504, -6.0575) -> (-20.3535, -6.0194)
  line L1176 (-20.3535, -6.0194) -> (-20.4993, -5.5022)
  line L1177 (-20.4993, -5.5022) -> (-20.346, -5.3637)
  line L1178 (-20.346, -5.3637) -> (-20.1392, -5.1861)
  line L1179 (-20.1392, -5.1861) -> (-19.9295, -5.0169)
  line L1180 (-19.9295, -5.0169) -> (-19.717, -4.8564)
  line L1181 (-19.717, -4.8564) -> (-19.5017, -4.7052)
  line L1182 (-19.5017, -4.7052) -> (-19.2836, -4.5639)
  line L1183 (-19.2836, -4.5639) -> (-19.0626, -4.4333)
  line L1184 (-19.0626, -4.4333) -> (-18.8385, -4.3147)
  line L1185 (-18.8385, -4.3147) -> (-18.7252, -4.2606)
  line L1186 (-18.7252, -4.2606) -> (-18.611, -4.2104)
  line L1187 (-18.611, -4.2104) -> (-18.4957, -4.1649)
  line L1188 (-18.4957, -4.1649) -> (-18.4376, -4.1443)
  line L1189 (-18.4376, -4.1443) -> (-18.379, -4.1257)
  line L1190 (-18.379, -4.1257) -> (-18.3791, -3.8359)
  line L1191 (-18.3791, -3.8359) -> (-18.448, -3.4895)
  line L1192 (-18.448, -3.4895) -> (-18.5588, -3.2217)
  line L1193 (-18.5588, -3.2217) -> (-18.62, -3.2269)
  line L1194 (-18.62, -3.2269) -> (-18.6816, -3.2301)
  line L1195 (-18.6816, -3.2301) -> (-18.8056, -3.2322)
  line L1196 (-18.8056, -3.2322) -> (-18.9303, -3.2296)
  line L1197 (-18.9303, -3.2296) -> (-19.0557, -3.2229)
  line L1198 (-19.0557, -3.2229) -> (-19.3081, -3.1991)
  line L1199 (-19.3081, -3.1991) -> (-19.5622, -3.163)
  line L1200 (-19.5622, -3.163) -> (-19.8178, -3.1159)
  line L1201 (-19.8178, -3.1159) -> (-20.0746, -3.0586)
  line L1202 (-20.0746, -3.0586) -> (-20.3323, -2.9917)
  line L1203 (-20.3323, -2.9917) -> (-20.5908, -2.9156)
  line L1204 (-20.5908, -2.9156) -> (-20.8499, -2.8307)
  line L1205 (-20.8499, -2.8307) -> (-21.0445, -2.7613)
  line L1206 (-21.0445, -2.7613) -> (-21.1077, -2.2277)
  line L1207 (-21.1077, -2.2277) -> (-20.9346, -2.1148)
  line L1208 (-20.9346, -2.1148) -> (-20.7025, -1.9718)
  line L1209 (-20.7025, -1.9718) -> (-20.4689, -1.8374)
  line L1210 (-20.4689, -1.8374) -> (-20.2339, -1.7122)
  line L1211 (-20.2339, -1.7122) -> (-19.9976, -1.5965)
  line L1212 (-19.9976, -1.5965) -> (-19.7601, -1.4911)
  line L1213 (-19.7601, -1.4911) -> (-19.5214, -1.3967)
  line L1214 (-19.5214, -1.3967) -> (-19.2815, -1.3146)
  line L1215 (-19.2815, -1.3146) -> (-19.1612, -1.2789)
  line L1216 (-19.1612, -1.2789) -> (-19.0405, -1.2472)
  line L1217 (-19.0405, -1.2472) -> (-18.9195, -1.2203)
  line L1218 (-18.9195, -1.2203) -> (-18.8589, -1.209)
  line L1219 (-18.8589, -1.209) -> (-18.7981, -1.1998)
  line L1220 (-18.7981, -1.1998) -> (-18.7529, -0.9135)
  line L1221 (-18.7529, -0.9135) -> (-18.7667, -0.5606)
  circle A19 centre (0, 0) radius 0.5
  line L1222 (-21.2068, 0.8332) -> (21.2068, -0.8332) construction
  line L1223 (-0.8332, -21.2068) -> (0.8332, 21.2068) construction
  dimension "d33" = 1
  dimension "d36" = 360
  dimension "d43" = 2.25
  constraints: 41 point on circle, 36 end point, 18 centre point, 4 coincident, 4 collinear, 2 concentric, 1 horizontal, 1 vertical, 76 other
extrude "Extrusion9" add sketch "Sketch10" along normal mid plane 5 contours A0 L16 A4 L17 | L15 A4 L14 A0 | A0 L19 A4 L18 | L12 A4 L13 A0 | A0 L20 A4 L21 | L11 A4 L10 A0 | A0 L3 A2 L2 | L7 A3 L6 A0 | L22 L23 L24 L25 L26 L27 L28 L29 L30 L31 L32 L33 L34 L35 L36 L37 L38 L39 L40 L41 L42 L43 L44 L45 L46 L47 L48 L49 L50 L51 L52 L53 L54 L55 L56 L57 L58 L59 L60 L61 L62 L63 L64 L65 L66 L67 L68 L69 L70 L71 L72 L73 L74 L75 L76 L77 L78 L79 L80 L81 L82 L83 L84 L85 L86 L87 L88 L89 L90 L91 L92 L93 L94 L95 L96 L97 L98 L99 L100 L101 L102 L103 L104 L105 L106 L107 L108 L109 L110 L111 L112 L113 L114 L115 L116 L117 L118 L119 L120 L121 L122 L123 L124 L125 L126 L127 L128 L129 L130 L131 L132 L133 L134 L135 L136 L137 L138 L139 L140 L141 L142 L143 L144 L145 L146 L147 L148 L149 L150 L151 L152 L153 L154 L155 L156 L157 L158 L159 L160 L161 L162 L163 L164 L165 L166 L167 L168 L169 L170 L171 L172 L173 L174 L175 L176 L177 L178 L179 L180 L181 L182 L183 L184 L185 L186 L187 L188 L189 L190 L191 L192 L193 L194 L195 L196 L197 L198 L199 L200 L201 L202 L203 L204 L205 L206 L207 L208 L209 L210 L211 L212 L213 L214 L215 L216 L217 L218 L219 L220 L221 L222 L223 L224 L225 L226 L227 L228 L229 L230 L231 L232 L233 L234 L235 L236 L237 L238 L239 L240 L241 L242 L243 L244 L245 L246 L247 L248 L249 L250 L251 L252 L253 L254 L255 L256 L257 L258 L259 L260 L261 L262 L263 L264 L265 L266 L267 L268 L269 L270 L271 L272 L273 L274 L275 L276 L277 L278 L279 L280 L281 L282 L283 L284 L285 L286 L287 L288 L289 L290 L291 L292 L293 L294 L295 L296 L297 L298 L299 L300 L301 L302 L303 L304 L305 L306 L307 L308 L309 L310 L311 L312 L313 L314 L315 L316 L317 L318 L319 L320 L321 L322 L323 L324 L325 L326 L327 L328 L329 L330 L331 L332 L333 L334 L335 L336 L337 L338 L339 L340 L341 L342 L343 L344 L345 L346 L347 L348 L349 L350 L351 L352 L353 L354 L355 L356 L357 L358 L359 L360 L361 L362 L363 L364 L365 L366 L367 L368 L369 L370 L371 L372 L373 L374 L375 L376 L377 L378 L379 L380 L381 L382 L383 L384 L385 L386 L387 L388 L389 L390 L391 L392 L393 L394 L395 L396 L397 L398 L399 L400 L401 L402 L403 L404 L405 L406 L407 L408 L409 L410 L411 L412 L413 L414 L415 L416 L417 L418 L419 L420 L421 L422 L423 L424 L425 L426 L427 L428 L429 L430 L431 L432 L433 L434 L435 L436 L437 L438 L439 L440 L441 L442 L443 L444 L445 L446 L447 L448 L449 L450 L451 L452 L453 L454 L455 L456 L457 L458 L459 L460 L461 L462 L463 L464 L465 L466 L467 L468 L469 L470 L471 L472 L473 L474 L475 L476 L477 L478 L479 L480 L481 L482 L483 L484 L485 L486 L487 L488 L489 L490 L491 L492 L493 L494 L495 L496 L497 L498 L499 L500 L501 L502 L503 L504 L505 L506 L507 L508 L509 L510 L511 L512 L513 L514 L515 L516 L517 L518 L519 L520 L521 L522 L523 L524 L525 L526 L527 L528 L529 L530 L531 L532 L533 L534 L535 L536 L537 L538 L539 L540 L541 L542 L543 L544 L545 L546 L547 L548 L549 L550 L551 L552 L553 L554 L555 L556 L557 L558 L559 L560 L561 L562 L563 L564 L565 L566 L567 L568 L569 L570 L571 L572 L573 L574 L575 L576 L577 L578 L579 L580 L581 L582 L583 L584 L585 L586 L587 L588 L589 L590 L591 L592 L593 L594 L595 L596 L597 L598 L599 L600 L601 L602 L603 L604 L605 L606 L607 L608 L609 L610 L611 L612 L613 L614 L615 L616 L617 L618 L619 L620 L621 L622 L623 L624 L625 L626 L627 L628 L629 L630 L631 L632 L633 L634 L635 L636 L637 L638 L639 L640 L641 L642 L643 L644 L645 L646 L647 L648 L649 L650 L651 L652 L653 L654 L655 L656 L657 L658 L659 L660 L661 L662 L663 L664 L665 L666 L667 L668 L669 L670 L671 L672 L673 L674 L675 L676 L677 L678 L679 L680 L681 L682 L683 L684 L685 L686 L687 L688 L689 L690 L691 L692 L693 L694 L695 L696 L697 L698 L699 L700 L701 L702 L703 L704 L705 L706 L707 L708 L709 L710 L711 L712 L713 L714 L715 L716 L717 L718 L719 L720 L721 L722 L723 L724 L725 L726 L727 L728 L729 L730 L731 L732 L733 L734 L735 L736 L737 L738 L739 L740 L741 L742 L743 L744 L745 L746 L747 L748 L749 L750 L751 L752 L753 L754 L755 L756 L757 L758 L759 L760 L761 L762 L763 L764 L765 L766 L767 L768 L769 L770 L771 L772 L773 L774 L775 L776 L777 L778 L779 L780 L781 L782 L783 L784 L785 L786 L787 L788 L789 L790 L791 L792 L793 L794 L795 L796 L797 L798 L799 L800 L801 L802 L803 L804 L805 L806 L807 L808 L809 L810 L811 L812 L813 L814 L815 L816 L817 L818 L819 L820 L821 L822 L823 L824 L825 L826 L827 L828 L829 L830 L831 L832 L833 L834 L835 L836 L837 L838 L839 L840 L841 L842 L843 L844 L845 L846 L847 L848 L849 L850 L851 L852 L853 L854 L855 L856 L857 L858 L859 L860 L861 L862 L863 L864 L865 L866 L867 L868 L869 L870 L871 L872 L873 L874 L875 L876 L877 L878 L879 L880 L881 L882 L883 L884 L885 L886 L887 L888 L889 L890 L891 L892 L893 L894 L895 L896 L897 L898 L899 L900 L901 L902 L903 L904 L905 L906 L907 L908 L909 L910 L911 L912 L913 L914 L915 L916 L917 L918 L919 L920 L921 L922 L923 L924 L925 L926 L927 L928 L929 L930 L931 L932 L933 L934 L935 L936 L937 L938 L939 L940 L941 L942 L943 L944 L945 L946 L947 L948 L949 L950 L951 L952 L953 L954 L955 L956 L957 L958 L959 L960 L961 L962 L963 L964 L965 L966 L967 L968 L969 L970 L971 L972 L973 L974 L975 L976 L977 L978 L979 L980 L981 L982 L983 L984 L985 L986 L987 L988 L989 L990 L991 L992 L993 L994 L995 L996 L997 L998 L999 L1000 L1001 L1002 L1003 L1004 L1005 L1006 L1007 L1008 L1009 L1010 L1011 L1012 L1013 L1014 L1015 L1016 L1017 L1018 L1019 L1020 L1021 L1022 L1023 L1024 L1025 L1026 L1027 L1028 L1029 L1030 L1031 L1032 L1033 L1034 L1035 L1036 L1037 L1038 L1039 L1040 L1041 L1042 L1043 L1044 L1045 L1046 L1047 L1048 L1049 L1050 L1051 L1052 L1053 L1054 L1055 L1056 L1057 L1058 L1059 L1060 L1061 L1062 L1063 L1064 L1065 L1066 L1067 L1068 L1069 L1070 L1071 L1072 L1073 L1074 L1075 L1076 L1077 L1078 L1079 L1080 L1081 L1082 L1083 L1084 L1085 L1086 L1087 L1088 L1089 L1090 L1091 L1092 L1093 L1094 L1095 L1096 L1097 L1098 L1099 L1100 L1101 L1102 L1103 L1104 L1105 L1106 L1107 L1108 L1109 L1110 L1111 L1112 L1113 L1114 L1115 L1116 L1117 L1118 L1119 L1120 L1121 L1122 L1123 L1124 L1125 L1126 L1127 L1128 L1129 L1130 L1131 L1132 L1133 L1134 L1135 L1136 L1137 L1138 L1139 L1140 L1141 L1142 L1143 L1144 L1145 L1146 L1147 L1148 L1149 L1150 L1151 L1152 L1153 L1154 L1155 L1156 L1157 L1158 L1159 L1160 L1161 L1162 L1163 L1164 L1165 L1166 L1167 L1168 L1169 L1170 L1171 L1172 L1173 L1174 L1175 L1176 L1177 L1178 L1179 L1180 L1181 L1182 L1183 L1184 L1185 L1186 L1187 L1188 L1189 L1190 L1191 L1192 L1193 L1194 L1195 L1196 L1197 L1198 L1199 L1200 L1201 L1202 L1203 L1204 L1205 L1206 L1207 L1208 L1209 L1210 L1211 L1212 L1213 L1214 L1215 L1216 L1217 L1218 L1219 L1220 L1221
extrude "Extrusion10" add sketch "Sketch10" along normal mid plane 1 contours A0 L17 A4 L15 | A0 L18 A4 L16 | L14 A4 L12 A0 | A0 L21 A4 L19 | L13 A4 L11 A0 | A0 L2 A4 L20 | L10 A4 L7 A0 | A0 L6 A1 L3
body "Solid4"
